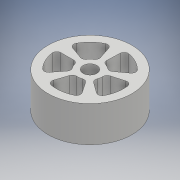
# Autodesk Inventor part: Rueda_Rin
Saved by Autodesk Inventor 2017 (Build 210142000, 142)
## iProperties
Created: 2016-07-28
Part Number: Rueda_Rin
Material: Generic
Document SubType Name: Modeling
Designer: ANDRES
Density: 1 g/cm^3
Appearance: Default
Author: ANDRES
## iProperties of the stored document Rueda_Rin_3DPrint.ipt
Created: 2016-09-14
Part Number: Rueda_Rin_3DPrint
Material: Generic
Document SubType Name: Modeling
Designer: ANDRES
Density: 1 g/cm^3
Appearance: Default
Author: ANDRES
Autodesk Inventor part; units mm, degrees
ref_plane "YZ Plane" through (0, 0, 0) normal (1, 0, 0) x (0, 1, 0)
ref_plane "XZ Plane" through (0, 0, 0) normal (0, 1, 0) x (-1, 0, 0)
ref_plane "XY Plane" through (0, 0, 0) normal (0, 0, 1) x (1, 0, 0)
sketch "Sketch4" plane through (0, 0, 0) normal (0, 0, 1) x (1, 0, 0)
  circle A0 centre (0, 0) radius 10
  arc A1 (-0.309, 0.9511) -> (-0.6428, 0.766) centre (0, 0) ccw
  line L0 (0, 0) -> (-0.309, 0.9511) construction
  line L1 (0, 0) -> (-0.9397, 0.342) construction
  arc A2 (0.5592, 0.829) -> (-0.309, 0.9511) centre (0, 0) ccw
  line L2 (-6.5104, 2.3696) -> (-2.8191, 1.0261)
  line L3 (-2.1409, 6.5891) -> (-0.9271, 2.8532)
  line L4 (-2.8191, 1.0261) -> (-6.5104, 2.3696)
  line L5 (-0.9271, 2.8532) -> (-2.1409, 6.5891)
  line L6 (-3, 0) -> (-6.9282, 0)
  arc A3 (-0.9397, 0.342) -> (-1, 0) centre (0, 0) ccw
  arc A4 (-0.309, 0.9511) -> (-0.9397, 0.342) centre (0, 0) ccw
  arc A5 (0.0349, 0.9994) -> (-0.309, 0.9511) centre (0, 0) ccw
  line L7 (0, 0) -> (0.0349, 0.9994) construction
  line L8 (0, 0) -> (-0.309, 0.9511) construction
  arc A6 (0.809, 0.5878) -> (0.0349, 0.9994) centre (0, 0) ccw
  line L9 (0, 0) -> (0.809, 0.5878) construction
  line L10 (0, 0) -> (0.0349, 0.9994) construction
  arc A7 (0.9613, 0.2756) -> (0.809, 0.5878) centre (0, 0) ccw
  line L11 (0, 0) -> (0.9613, 0.2756) construction
  line L12 (0, 0) -> (0.809, 0.5878) construction
  arc A8 (0.809, -0.5878) -> (0.9613, 0.2756) centre (0, 0) ccw
  line L13 (0, 0) -> (0.809, -0.5878) construction
  line L14 (0, 0) -> (0.9613, 0.2756) construction
  arc A9 (0.5592, -0.829) -> (0.809, -0.5878) centre (0, 0) ccw
  line L15 (0, 0) -> (0.5592, -0.829) construction
  line L16 (0, 0) -> (0.809, -0.5878) construction
  arc A10 (-0.309, -0.9511) -> (0.5592, -0.829) centre (0, 0) ccw
  line L17 (0, 0) -> (-0.309, -0.9511) construction
  line L18 (0, 0) -> (0.5592, -0.829) construction
  arc A11 (-0.6157, -0.788) -> (-0.309, -0.9511) centre (0, 0) ccw
  line L19 (0, 0) -> (-0.6157, -0.788) construction
  line L20 (0, 0) -> (-0.309, -0.9511) construction
  arc A12 (-1, 0) -> (-0.6157, -0.788) centre (0, 0) ccw
  line L21 (0.1047, 2.9982) -> (0.2418, 6.924) construction
  line L22 (-1.847, -2.364) -> (-4.2654, -5.4595) construction
  line L23 (-1.847, -2.364) -> (-4.2654, -5.4595)
  line L24 (-0.9271, -2.8532) -> (-2.1409, -6.5891)
  line L25 (1.6776, -2.4871) -> (3.8742, -5.7437)
  line L26 (2.4271, -1.7634) -> (5.605, -4.0723)
  line L27 (2.8838, 0.8269) -> (6.6598, 1.9097)
  line L28 (2.4271, 1.7634) -> (5.605, 4.0723)
  line L29 (0.1047, 2.9982) -> (0.2418, 6.924)
  arc A13 (-1.8794, 0.684) -> (-2, 0) centre (0, 0) ccw
  line L30 (0, 0) -> (0.809, 0.5878) construction
  line L31 (2.4271, 1.7634) -> (5.605, 4.0723) construction
  line L32 (0, 0) -> (-0.309, 0.9511) construction
  line L33 (-0.9271, 2.8532) -> (-2.3011, 7.0821) construction
  line L34 (0, 0) -> (0.0349, 0.9994) construction
  line L35 (0.1047, 2.9982) -> (0.2418, 6.924) construction
  line L36 (0, 0) -> (-0.309, 0.9511) construction
  line L37 (-0.9271, 2.8532) -> (-2.3011, 7.0821) construction
  line L38 (-1.6276, 0.5924) -> (-1.8794, 0.684) construction
  line L39 (-2.8191, 1.0261) -> (-6.9975, 2.5469) construction
  line L40 (0, 0) -> (-0.309, -0.9511) construction
  line L41 (-0.9271, -2.8532) -> (-2.1409, -6.5891) construction
  line L42 (0, 0) -> (0.5592, -0.829) construction
  line L43 (1.6776, -2.4871) -> (3.8742, -5.7437) construction
  line L44 (0, 0) -> (0.809, -0.5878) construction
  line L45 (2.4271, -1.7634) -> (6.0244, -4.377) construction
  line L46 (0, 0) -> (0.9613, 0.2756) construction
  line L47 (2.8838, 0.8269) -> (6.6598, 1.9097) construction
  line L48 (0, 0) -> (-0.309, -0.9511) construction
  line L49 (-0.9271, -2.8532) -> (-2.3011, -7.0821) construction
  line L50 (0, 0) -> (0.5592, -0.829) construction
  line L51 (1.5816, -2.3449) -> (3.8742, -5.7437) construction
  line L52 (0, 0) -> (0.9613, 0.2756) construction
  line L53 (2.8838, 0.8269) -> (7.1581, 2.0526) construction
  arc A14 (-1.3599, -7.8836) -> (3.4802, -7.2034) centre (0, 0) ccw
  arc A15 (-7.9179, -1.1429) -> (-5.7754, -5.5358) centre (0, 0) ccw
  arc A16 (-3.5337, 7.1773) -> (-7.0496, 3.782) centre (0, 0) ccw
  arc A17 (5.734, 5.5786) -> (1.4185, 7.8732) centre (0, 0) ccw
  arc A18 (7.0775, -3.7295) -> (7.9262, 1.0839) centre (0, 0) ccw
  arc A19 (5.605, -4.0723) -> (7.0775, -3.7295) centre (6.1928, -3.2633) ccw
  arc A20 (7.9262, 1.0839) -> (6.6598, 1.9097) centre (6.9355, 0.9484) ccw
  arc A21 (5.605, 4.0723) -> (5.734, 5.5786) centre (5.0172, 4.8813) ccw
  arc A22 (1.4185, 7.8732) -> (0.2418, 6.924) centre (1.2412, 6.8891) ccw
  arc A23 (-2.1409, 6.5891) -> (-3.5337, 7.1773) centre (-3.092, 6.2801) ccw
  arc A24 (-7.0496, 3.782) -> (-6.5104, 2.3696) centre (-6.1684, 3.3093) ccw
  arc A25 (-6.9282, 0) -> (-7.9179, -1.1429) centre (-6.9282, -1) ccw
  arc A26 (-5.7754, -5.5358) -> (-4.2654, -5.4595) centre (-5.0534, -4.8438) ccw
  arc A27 (-2.1409, -6.5891) -> (-1.3599, -7.8836) centre (-1.1899, -6.8981) ccw
  arc A28 (3.4802, -7.2034) -> (3.8742, -5.7437) centre (3.0452, -6.3029) ccw
  circle A29 centre (0, 0) radius 3
  line L54 (0, 0) -> (-0.309, 0.9511) construction
  line L55 (-0.9271, 2.8532) -> (-2.1409, 6.5891) construction
  line L56 (0, 0) -> (0.809, 0.5878) construction
  line L57 (2.4271, 1.7634) -> (5.605, 4.0723) construction
  line L58 (-0.809, 0.5878) -> (0.809, -0.5878) construction
  line L59 (2.4271, -1.7634) -> (5.605, -4.0723) construction
  point P0 (-4.5846, -5.868)
  point P1 (-1.7414, -2.2288)
  dimension "d123" = 6
  dimension "d33" = 20
  dimension "d42" = 52
  dimension "d50" = 20
  dimension "d51" = 52
  dimension "d52" = 20
  dimension "d53" = 52
  dimension "d54" = 20
  dimension "d55" = 52
  dimension "d56" = 20
  dimension "d65" = 2
  dimension "d77" = 8
  dimension "d78" = 1
  constraints: 90 end point, 41 point on circle, 21 centre point, 21 tangent, 17 point on line, 9 equal radius, 2 collinear, 1 coincident, 1 horizontal, 75 other
  measures "d33" diameter of A0
  measures "d42" angle of L0 L1
  measures "d50" angle of L7 L8
  measures "d51" angle of L9 L10
  measures "d52" angle of L11 L12
  measures "d53" angle of L13 L14
  measures "d54" angle of L15 L16
  measures "d55" angle of L17 L18
  measures "d56" angle of L19 L20
  measures "d65" radius of A13
  measures "d77" radius of A14
  measures "d78" radius of A19
extrude "Extrusion9" add sketch "Sketch4" along normal blind 8.5 contours A0 | A29
sketch "Engranaje41" plane through (0, 0, 0) normal (0, 0, -1) x (-1, 0, 0)
  circle A0 centre (0, 0) radius 1
  arc A1 (1.256, 9.9788) -> (1.0973, 10.6734) centre (-2.5912, 9.4651) ccw
  arc A2 (1.0973, 10.6734) -> (0.854, 10.6956) centre (0, 0) ccw
  arc A3 (0.854, 10.6956) -> (0.5721, 10.0412) centre (4.2626, 8.8392) ccw
  arc A4 (0.5721, 10.0412) -> (0.3434, 10.0517) centre (0, 0) ccw
  arc A5 (0.3434, 10.0517) -> (0.1221, 10.729) centre (-3.4411, 9.1902) ccw
  arc A6 (0.1221, 10.729) -> (-0.1221, 10.729) centre (0, 0) ccw
  arc A7 (-0.1221, 10.729) -> (-0.3434, 10.0517) centre (3.4411, 9.1902) ccw
  arc A8 (-0.3434, 10.0517) -> (-0.5721, 10.0412) centre (0, 0) ccw
  arc A9 (-0.5721, 10.0412) -> (-0.854, 10.6956) centre (-4.2626, 8.8392) ccw
  arc A10 (-0.854, 10.6956) -> (-1.0973, 10.6734) centre (0, 0) ccw
  arc A11 (-1.0973, 10.6734) -> (-1.256, 9.9788) centre (2.5912, 9.4651) ccw
  arc A12 (-1.256, 9.9788) -> (-1.4828, 9.9476) centre (0, 0) ccw
  arc A13 (-1.4828, 9.9476) -> (-1.8231, 10.5737) centre (-5.0487, 8.415) ccw
  arc A14 (-1.8231, 10.5737) -> (-2.0633, 10.5294) centre (0, 0) ccw
  arc A15 (-2.0633, 10.5294) -> (-2.1582, 9.8232) centre (1.7197, 9.6615) ccw
  arc A16 (-2.1582, 9.8232) -> (-2.3813, 9.7716) centre (0, 0) ccw
  arc A17 (-2.3813, 9.7716) -> (-2.777, 10.3641) centre (-5.793, 7.921) ccw
  arc A18 (-2.777, 10.3641) -> (-3.0122, 10.2982) centre (0, 0) ccw
  arc A19 (-3.0122, 10.2982) -> (-3.0425, 9.5863) centre (0.834, 9.7778) ccw
  arc A20 (-3.0425, 9.5863) -> (-3.26, 9.5145) centre (0, 0) ccw
  arc A21 (-3.26, 9.5145) -> (-3.708, 10.0686) centre (-6.4893, 7.3614) ccw
  arc A22 (-3.708, 10.0686) -> (-3.9362, 9.9816) centre (0, 0) ccw
  arc A23 (-3.9362, 9.9816) -> (-3.9017, 9.2699) centre (-0.0586, 9.8132) ccw
  arc A24 (-3.9017, 9.2699) -> (-4.1117, 9.1787) centre (0, 0) ccw
  arc A25 (-4.1117, 9.1787) -> (-4.6082, 9.6897) centre (-7.1318, 6.7408) ccw
  arc A26 (-4.6082, 9.6897) -> (-4.8276, 9.5823) centre (0, 0) ccw
  arc A27 (-4.8276, 9.5823) -> (-4.7285, 8.8767) centre (-0.9507, 9.7672) ccw
  arc A28 (-4.7285, 8.8767) -> (-4.9293, 8.7667) centre (0, 0) ccw
  arc A29 (-4.9293, 8.7667) -> (-5.4703, 9.2305) centre (-7.7153, 6.0644) ccw
  arc A30 (-5.4703, 9.2305) -> (-5.679, 9.1036) centre (0, 0) ccw
  arc A31 (-5.679, 9.1036) -> (-5.5161, 8.4099) centre (-1.8349, 9.6403) ccw
  arc A32 (-5.5161, 8.4099) -> (-5.7061, 8.2822) centre (0, 0) ccw
  arc A33 (-5.7061, 8.2822) -> (-6.287, 8.6948) centre (-8.2348, 5.3376) ccw
  arc A34 (-6.287, 8.6948) -> (-6.4833, 8.5495) centre (0, 0) ccw
  arc A35 (-6.4833, 8.5495) -> (-6.258, 7.8735) centre (-2.704, 9.4335) ccw
  arc A36 (-6.258, 7.8735) -> (-6.4356, 7.729) centre (0, 0) ccw
  arc A37 (-6.4356, 7.729) -> (-7.0516, 8.0871) centre (-8.686, 4.5667) ccw
  arc A38 (-7.0516, 8.0871) -> (-7.2338, 7.9245) centre (0, 0) ccw
  arc A39 (-7.2338, 7.9245) -> (-6.948, 7.2718) centre (-3.5506, 9.1485) ccw
  arc A40 (-6.948, 7.2718) -> (-7.1117, 7.1117) centre (0, 0) ccw
  arc A41 (-7.1117, 7.1117) -> (-7.7578, 7.4124) centre (-9.0653, 3.7579) ccw
  arc A42 (-7.7578, 7.4124) -> (-7.9245, 7.2338) centre (0, 0) ccw
  arc A43 (-7.9245, 7.2338) -> (-7.5805, 6.6098) centre (-4.3678, 8.7877) ccw
  arc A44 (-7.5805, 6.6098) -> (-7.729, 6.4356) centre (0, 0) ccw
  arc A45 (-7.729, 6.4356) -> (-8.3997, 6.6762) centre (-9.3695, 2.918) ccw
  arc A46 (-8.3997, 6.6762) -> (-8.5495, 6.4833) centre (0, 0) ccw
  arc A47 (-8.5495, 6.4833) -> (-8.1501, 5.8931) centre (-5.1488, 8.3541) ccw
  arc A48 (-8.1501, 5.8931) -> (-8.2822, 5.7061) centre (0, 0) ccw
  arc A49 (-8.2822, 5.7061) -> (-8.972, 5.8847) centre (-9.596, 2.0539) ccw
  arc A50 (-8.972, 5.8847) -> (-9.1036, 5.679) centre (0, 0) ccw
  arc A51 (-9.1036, 5.679) -> (-8.6523, 5.1276) centre (-5.8872, 7.8513) ccw
  arc A52 (-8.6523, 5.1276) -> (-8.7667, 4.9293) centre (0, 0) ccw
  arc A53 (-8.7667, 4.9293) -> (-9.4699, 5.0445) centre (-9.743, 1.1728) ccw
  arc A54 (-9.4699, 5.0445) -> (-9.5823, 4.8276) centre (0, 0) ccw
  arc A55 (-9.5823, 4.8276) -> (-9.0827, 4.3195) centre (-6.5767, 7.2834) ccw
  arc A56 (-9.0827, 4.3195) -> (-9.1787, 4.1117) centre (0, 0) ccw
  arc A57 (-9.1787, 4.1117) -> (-9.8894, 4.1624) centre (-9.8093, 0.2819) ccw
  arc A58 (-9.8894, 4.1624) -> (-9.9816, 3.9362) centre (0, 0) ccw
  arc A59 (-9.9816, 3.9362) -> (-9.4379, 3.4757) centre (-7.2118, 6.6552) ccw
  arc A60 (-9.4379, 3.4757) -> (-9.5145, 3.26) centre (0, 0) ccw
  arc A61 (-9.5145, 3.26) -> (-10.2269, 3.2459) centre (-9.7943, -0.6112) ccw
  arc A62 (-10.2269, 3.2459) -> (-10.2982, 3.0122) centre (0, 0) ccw
  arc A63 (-10.2982, 3.0122) -> (-9.7148, 2.6031) centre (-7.7871, 5.9718) ccw
  arc A64 (-9.7148, 2.6031) -> (-9.7716, 2.3813) centre (0, 0) ccw
  arc A65 (-9.7716, 2.3813) -> (-10.4797, 2.3024) centre (-9.6981, -1.4994) ccw
  arc A66 (-10.4797, 2.3024) -> (-10.5294, 2.0633) centre (0, 0) ccw
  arc A67 (-10.5294, 2.0633) -> (-9.9113, 1.7089) centre (-8.2979, 5.239) ccw
  arc A68 (-9.9113, 1.7089) -> (-9.9476, 1.4828) centre (0, 0) ccw
  arc A69 (-9.9476, 1.4828) -> (-10.6457, 1.3399) centre (-9.5216, -2.375) ccw
  arc A70 (-10.6457, 1.3399) -> (-10.6734, 1.0973) centre (0, 0) ccw
  arc A71 (-10.6734, 1.0973) -> (-10.0256, 0.8005) centre (-8.7399, 4.4627) ccw
  arc A72 (-10.0256, 0.8005) -> (-10.0412, 0.5721) centre (0, 0) ccw
  arc A73 (-10.0412, 0.5721) -> (-10.7234, 0.3663) centre (-9.2662, -3.231) ccw
  arc A74 (-10.7234, 0.3663) -> (-10.729, 0.1221) centre (0, 0) ccw
  arc A75 (-10.729, 0.1221) -> (-10.0569, -0.1145) centre (-9.1095, 3.6494) ccw
  arc A76 (-10.0569, -0.1145) -> (-10.0517, -0.3434) centre (0, 0) ccw
  arc A77 (-10.0517, -0.3434) -> (-10.7123, -0.6103) centre (-8.934, -4.0603) ccw
  arc A78 (-10.7123, -0.6103) -> (-10.6956, -0.854) centre (0, 0) ccw
  arc A79 (-10.6956, -0.854) -> (-10.0048, -1.0285) centre (-9.4036, 2.806) ccw
  arc A80 (-10.0048, -1.0285) -> (-9.9788, -1.256) centre (0, 0) ccw
  arc A81 (-9.9788, -1.256) -> (-10.6124, -1.5819) centre (-8.5277, -4.8559) ccw
  arc A82 (-10.6124, -1.5819) -> (-10.5737, -1.8231) centre (0, 0) ccw
  arc A83 (-10.5737, -1.8231) -> (-9.8698, -1.934) centre (-9.6198, 1.9392) ccw
  arc A84 (-9.8698, -1.934) -> (-9.8232, -2.1582) centre (0, 0) ccw
  arc A85 (-9.8232, -2.1582) -> (-10.4246, -2.5404) centre (-8.0508, -5.6112) ccw
  arc A86 (-10.4246, -2.5404) -> (-10.3641, -2.777) centre (0, 0) ccw
  arc A87 (-10.3641, -2.777) -> (-9.653, -2.8235) centre (-9.7563, 1.0564) ccw
  arc A88 (-9.653, -2.8235) -> (-9.5863, -3.0425) centre (0, 0) ccw
  arc A89 (-9.5863, -3.0425) -> (-10.1504, -3.4778) centre (-7.5072, -6.3201) ccw
  arc A90 (-10.1504, -3.4778) -> (-10.0686, -3.708) centre (0, 0) ccw
  arc A91 (-10.0686, -3.708) -> (-9.3563, -3.6896) centre (-9.812, 0.1648) ccw
  arc A92 (-9.3563, -3.6896) -> (-9.2699, -3.9017) centre (0, 0) ccw
  arc A93 (-9.2699, -3.9017) -> (-9.7921, -4.3865) centre (-6.9014, -6.9766) ccw
  arc A94 (-9.7921, -4.3865) -> (-9.6897, -4.6082) centre (0, 0) ccw
  arc A95 (-9.6897, -4.6082) -> (-8.982, -4.5252) centre (-9.7863, -0.7281) ccw
  arc A96 (-8.982, -4.5252) -> (-8.8767, -4.7285) centre (0, 0) ccw
  arc A97 (-8.8767, -4.7285) -> (-9.3526, -5.2587) centre (-6.2384, -7.5752) ccw
  arc A98 (-9.3526, -5.2587) -> (-9.2305, -5.4703) centre (0, 0) ccw
  arc A99 (-9.2305, -5.4703) -> (-8.5333, -5.3232) centre (-9.6795, -1.615) ccw
  arc A100 (-8.5333, -5.3232) -> (-8.4099, -5.5161) centre (0, 0) ccw
  arc A101 (-8.4099, -5.5161) -> (-8.8357, -6.0874) centre (-5.5237, -8.1111) ccw
  arc A102 (-8.8357, -6.0874) -> (-8.6948, -6.287) centre (0, 0) ccw
  arc A103 (-8.6948, -6.287) -> (-8.0139, -6.0771) centre (-9.4926, -2.4885) ccw
  arc A104 (-8.0139, -6.0771) -> (-7.8735, -6.258) centre (0, 0) ccw
  arc A105 (-7.8735, -6.258) -> (-8.2455, -6.8657) centre (-4.7632, -8.5798) ccw
  arc A106 (-8.2455, -6.8657) -> (-8.0871, -7.0516) centre (0, 0) ccw
  arc A107 (-8.0871, -7.0516) -> (-7.4281, -6.7807) centre (-9.227, -3.3414) ccw
  arc A108 (-7.4281, -6.7807) -> (-7.2718, -6.948) centre (0, 0) ccw
  arc A109 (-7.2718, -6.948) -> (-7.587, -7.587) centre (-3.9633, -8.9774) ccw
  arc A110 (-7.587, -7.587) -> (-7.4124, -7.7578) centre (0, 0) ccw
  arc A111 (-7.4124, -7.7578) -> (-6.7807, -7.4281) centre (-8.8849, -4.1666) ccw
  arc A112 (-6.7807, -7.4281) -> (-6.6098, -7.5805) centre (0, 0) ccw
  arc A113 (-6.6098, -7.5805) -> (-6.8657, -8.2455) centre (-3.1305, -9.3006) ccw
  arc A114 (-6.8657, -8.2455) -> (-6.6762, -8.3997) centre (0, 0) ccw
  arc A115 (-6.6762, -8.3997) -> (-6.0771, -8.0139) centre (-8.4692, -4.9573) ccw
  arc A116 (-6.0771, -8.0139) -> (-5.8931, -8.1501) centre (0, 0) ccw
  arc A117 (-5.8931, -8.1501) -> (-6.0874, -8.8357) centre (-2.2718, -9.5468) ccw
  arc A118 (-6.0874, -8.8357) -> (-5.8847, -8.972) centre (0, 0) ccw
  arc A119 (-5.8847, -8.972) -> (-5.3232, -8.5333) centre (-7.9833, -5.7069) ccw
  arc A120 (-5.3232, -8.5333) -> (-5.1276, -8.6523) centre (0, 0) ccw
  arc A121 (-5.1276, -8.6523) -> (-5.2587, -9.3526) centre (-1.3942, -9.7138) ccw
  arc A122 (-5.2587, -9.3526) -> (-5.0445, -9.4699) centre (0, 0) ccw
  arc A123 (-5.0445, -9.4699) -> (-4.5252, -8.982) centre (-7.4313, -6.4092) ccw
  arc A124 (-4.5252, -8.982) -> (-4.3195, -9.0827) centre (0, 0) ccw
  arc A125 (-4.3195, -9.0827) -> (-4.3865, -9.7921) centre (-0.5051, -9.8003) ccw
  arc A126 (-4.3865, -9.7921) -> (-4.1624, -9.8894) centre (0, 0) ccw
  arc A127 (-4.1624, -9.8894) -> (-3.6896, -9.3563) centre (-6.8177, -7.0584) ccw
  arc A128 (-3.6896, -9.3563) -> (-3.4757, -9.4379) centre (0, 0) ccw
  arc A129 (-3.4757, -9.4379) -> (-3.4778, -10.1504) centre (0.3881, -9.8057) ccw
  arc A130 (-3.4778, -10.1504) -> (-3.2459, -10.2269) centre (0, 0) ccw
  arc A131 (-3.2459, -10.2269) -> (-2.8235, -9.653) centre (-6.1475, -7.6492) ccw
  arc A132 (-2.8235, -9.653) -> (-2.6031, -9.7148) centre (0, 0) ccw
  arc A133 (-2.6031, -9.7148) -> (-2.5404, -10.4246) centre (1.2782, -9.7298) ccw
  arc A134 (-2.5404, -10.4246) -> (-2.3024, -10.4797) centre (0, 0) ccw
  arc A135 (-2.3024, -10.4797) -> (-1.934, -9.8698) centre (-5.4265, -8.1765) ccw
  arc A136 (-1.934, -9.8698) -> (-1.7089, -9.9113) centre (0, 0) ccw
  arc A137 (-1.7089, -9.9113) -> (-1.5819, -10.6124) centre (2.1577, -9.5732) ccw
  arc A138 (-1.5819, -10.6124) -> (-1.3399, -10.6457) centre (0, 0) ccw
  arc A139 (-1.3399, -10.6457) -> (-1.0285, -10.0048) centre (-4.6605, -8.6361) ccw
  arc A140 (-1.0285, -10.0048) -> (-0.8005, -10.0256) centre (0, 0) ccw
  arc A141 (-0.8005, -10.0256) -> (-0.6103, -10.7123) centre (3.0193, -9.3373) ccw
  arc A142 (-0.6103, -10.7123) -> (-0.3663, -10.7234) centre (0, 0) ccw
  arc A143 (-0.3663, -10.7234) -> (-0.1145, -10.0569) centre (-3.8559, -9.0241) ccw
  arc A144 (-0.1145, -10.0569) -> (0.1145, -10.0569) centre (0, 0) ccw
  arc A145 (0.1145, -10.0569) -> (0.3663, -10.7234) centre (3.8559, -9.0241) ccw
  arc A146 (0.3663, -10.7234) -> (0.6103, -10.7123) centre (0, 0) ccw
  arc A147 (0.6103, -10.7123) -> (0.8005, -10.0256) centre (-3.0193, -9.3373) ccw
  arc A148 (0.8005, -10.0256) -> (1.0285, -10.0048) centre (0, 0) ccw
  arc A149 (1.0285, -10.0048) -> (1.3399, -10.6457) centre (4.6605, -8.6361) ccw
  arc A150 (1.3399, -10.6457) -> (1.5819, -10.6124) centre (0, 0) ccw
  arc A151 (1.5819, -10.6124) -> (1.7089, -9.9113) centre (-2.1577, -9.5732) ccw
  arc A152 (1.7089, -9.9113) -> (1.934, -9.8698) centre (0, 0) ccw
  arc A153 (1.934, -9.8698) -> (2.3024, -10.4797) centre (5.4265, -8.1765) ccw
  arc A154 (2.3024, -10.4797) -> (2.5404, -10.4246) centre (0, 0) ccw
  arc A155 (2.5404, -10.4246) -> (2.6031, -9.7148) centre (-1.2782, -9.7298) ccw
  arc A156 (2.6031, -9.7148) -> (2.8235, -9.653) centre (0, 0) ccw
  arc A157 (2.8235, -9.653) -> (3.2459, -10.2269) centre (6.1475, -7.6492) ccw
  arc A158 (3.2459, -10.2269) -> (3.4778, -10.1504) centre (0, 0) ccw
  arc A159 (3.4778, -10.1504) -> (3.4757, -9.4379) centre (-0.3881, -9.8057) ccw
  arc A160 (3.4757, -9.4379) -> (3.6896, -9.3563) centre (0, 0) ccw
  arc A161 (3.6896, -9.3563) -> (4.1624, -9.8894) centre (6.8177, -7.0584) ccw
  arc A162 (4.1624, -9.8894) -> (4.3865, -9.7921) centre (0, 0) ccw
  arc A163 (4.3865, -9.7921) -> (4.3195, -9.0827) centre (0.5051, -9.8003) ccw
  arc A164 (4.3195, -9.0827) -> (4.5252, -8.982) centre (0, 0) ccw
  arc A165 (4.5252, -8.982) -> (5.0445, -9.4699) centre (7.4313, -6.4092) ccw
  arc A166 (5.0445, -9.4699) -> (5.2587, -9.3526) centre (0, 0) ccw
  arc A167 (5.2587, -9.3526) -> (5.1276, -8.6523) centre (1.3942, -9.7138) ccw
  arc A168 (5.1276, -8.6523) -> (5.3232, -8.5333) centre (0, 0) ccw
  arc A169 (5.3232, -8.5333) -> (5.8847, -8.972) centre (7.9833, -5.7069) ccw
  arc A170 (5.8847, -8.972) -> (6.0874, -8.8357) centre (0, 0) ccw
  arc A171 (6.0874, -8.8357) -> (5.8931, -8.1501) centre (2.2718, -9.5468) ccw
  arc A172 (5.8931, -8.1501) -> (6.0771, -8.0139) centre (0, 0) ccw
  arc A173 (6.0771, -8.0139) -> (6.6762, -8.3997) centre (8.4692, -4.9573) ccw
  arc A174 (6.6762, -8.3997) -> (6.8657, -8.2455) centre (0, 0) ccw
  arc A175 (6.8657, -8.2455) -> (6.6098, -7.5805) centre (3.1305, -9.3006) ccw
  arc A176 (6.6098, -7.5805) -> (6.7807, -7.4281) centre (0, 0) ccw
  arc A177 (6.7807, -7.4281) -> (7.4124, -7.7578) centre (8.8849, -4.1666) ccw
  arc A178 (7.4124, -7.7578) -> (7.587, -7.587) centre (0, 0) ccw
  arc A179 (7.587, -7.587) -> (7.2718, -6.948) centre (3.9633, -8.9774) ccw
  arc A180 (7.2718, -6.948) -> (7.4281, -6.7807) centre (0, 0) ccw
  arc A181 (7.4281, -6.7807) -> (8.0871, -7.0516) centre (9.227, -3.3414) ccw
  arc A182 (8.0871, -7.0516) -> (8.2455, -6.8657) centre (0, 0) ccw
  arc A183 (8.2455, -6.8657) -> (7.8735, -6.258) centre (4.7632, -8.5798) ccw
  arc A184 (7.8735, -6.258) -> (8.0139, -6.0771) centre (0, 0) ccw
  arc A185 (8.0139, -6.0771) -> (8.6948, -6.287) centre (9.4926, -2.4885) ccw
  arc A186 (8.6948, -6.287) -> (8.8357, -6.0874) centre (0, 0) ccw
  arc A187 (8.8357, -6.0874) -> (8.4099, -5.5161) centre (5.5237, -8.1111) ccw
  arc A188 (8.4099, -5.5161) -> (8.5333, -5.3232) centre (0, 0) ccw
  arc A189 (8.5333, -5.3232) -> (9.2305, -5.4703) centre (9.6795, -1.615) ccw
  arc A190 (9.2305, -5.4703) -> (9.3526, -5.2587) centre (0, 0) ccw
  arc A191 (9.3526, -5.2587) -> (8.8767, -4.7285) centre (6.2384, -7.5752) ccw
  arc A192 (8.8767, -4.7285) -> (8.982, -4.5252) centre (0, 0) ccw
  arc A193 (8.982, -4.5252) -> (9.6897, -4.6082) centre (9.7863, -0.7281) ccw
  arc A194 (9.6897, -4.6082) -> (9.7921, -4.3865) centre (0, 0) ccw
  arc A195 (9.7921, -4.3865) -> (9.2699, -3.9017) centre (6.9014, -6.9766) ccw
  arc A196 (9.2699, -3.9017) -> (9.3563, -3.6896) centre (0, 0) ccw
  arc A197 (9.3563, -3.6896) -> (10.0686, -3.708) centre (9.812, 0.1648) ccw
  arc A198 (10.0686, -3.708) -> (10.1504, -3.4778) centre (0, 0) ccw
  arc A199 (10.1504, -3.4778) -> (9.5863, -3.0425) centre (7.5072, -6.3201) ccw
  arc A200 (9.5863, -3.0425) -> (9.653, -2.8235) centre (0, 0) ccw
  arc A201 (9.653, -2.8235) -> (10.3641, -2.777) centre (9.7563, 1.0564) ccw
  arc A202 (10.3641, -2.777) -> (10.4246, -2.5404) centre (0, 0) ccw
  arc A203 (10.4246, -2.5404) -> (9.8232, -2.1582) centre (8.0508, -5.6112) ccw
  arc A204 (9.8232, -2.1582) -> (9.8698, -1.934) centre (0, 0) ccw
  arc A205 (9.8698, -1.934) -> (10.5737, -1.8231) centre (9.6198, 1.9392) ccw
  arc A206 (10.5737, -1.8231) -> (10.6124, -1.5819) centre (0, 0) ccw
  arc A207 (10.6124, -1.5819) -> (9.9788, -1.256) centre (8.5277, -4.8559) ccw
  arc A208 (9.9788, -1.256) -> (10.0048, -1.0285) centre (0, 0) ccw
  arc A209 (10.0048, -1.0285) -> (10.6956, -0.854) centre (9.4036, 2.806) ccw
  arc A210 (10.6956, -0.854) -> (10.7123, -0.6103) centre (0, 0) ccw
  arc A211 (10.7123, -0.6103) -> (10.0517, -0.3434) centre (8.934, -4.0603) ccw
  arc A212 (10.0517, -0.3434) -> (10.0569, -0.1145) centre (0, 0) ccw
  arc A213 (10.0569, -0.1145) -> (10.729, 0.1221) centre (9.1095, 3.6494) ccw
  arc A214 (10.729, 0.1221) -> (10.7234, 0.3663) centre (0, 0) ccw
  arc A215 (10.7234, 0.3663) -> (10.0412, 0.5721) centre (9.2662, -3.231) ccw
  arc A216 (10.0412, 0.5721) -> (10.0256, 0.8005) centre (0, 0) ccw
  arc A217 (10.0256, 0.8005) -> (10.6734, 1.0973) centre (8.7399, 4.4627) ccw
  arc A218 (10.6734, 1.0973) -> (10.6457, 1.3399) centre (0, 0) ccw
  arc A219 (10.6457, 1.3399) -> (9.9476, 1.4828) centre (9.5216, -2.375) ccw
  arc A220 (9.9476, 1.4828) -> (9.9113, 1.7089) centre (0, 0) ccw
  arc A221 (9.9113, 1.7089) -> (10.5294, 2.0633) centre (8.2979, 5.239) ccw
  arc A222 (10.5294, 2.0633) -> (10.4797, 2.3024) centre (0, 0) ccw
  arc A223 (10.4797, 2.3024) -> (9.7716, 2.3813) centre (9.6981, -1.4994) ccw
  arc A224 (9.7716, 2.3813) -> (9.7148, 2.6031) centre (0, 0) ccw
  arc A225 (9.7148, 2.6031) -> (10.2982, 3.0122) centre (7.7871, 5.9718) ccw
  arc A226 (10.2982, 3.0122) -> (10.2269, 3.2459) centre (0, 0) ccw
  arc A227 (10.2269, 3.2459) -> (9.5145, 3.26) centre (9.7943, -0.6112) ccw
  arc A228 (9.5145, 3.26) -> (9.4379, 3.4757) centre (0, 0) ccw
  arc A229 (9.4379, 3.4757) -> (9.9816, 3.9362) centre (7.2118, 6.6552) ccw
  arc A230 (9.9816, 3.9362) -> (9.8894, 4.1624) centre (0, 0) ccw
  arc A231 (9.8894, 4.1624) -> (9.1787, 4.1117) centre (9.8093, 0.2819) ccw
  arc A232 (9.1787, 4.1117) -> (9.0827, 4.3195) centre (0, 0) ccw
  arc A233 (9.0827, 4.3195) -> (9.5823, 4.8276) centre (6.5767, 7.2834) ccw
  arc A234 (9.5823, 4.8276) -> (9.4699, 5.0445) centre (0, 0) ccw
  arc A235 (9.4699, 5.0445) -> (8.7667, 4.9293) centre (9.743, 1.1728) ccw
  arc A236 (8.7667, 4.9293) -> (8.6523, 5.1276) centre (0, 0) ccw
  arc A237 (8.6523, 5.1276) -> (9.1036, 5.679) centre (5.8872, 7.8513) ccw
  arc A238 (9.1036, 5.679) -> (8.972, 5.8847) centre (0, 0) ccw
  arc A239 (8.972, 5.8847) -> (8.2822, 5.7061) centre (9.596, 2.0539) ccw
  arc A240 (8.2822, 5.7061) -> (8.1501, 5.8931) centre (0, 0) ccw
  arc A241 (8.1501, 5.8931) -> (8.5495, 6.4833) centre (5.1488, 8.3541) ccw
  arc A242 (8.5495, 6.4833) -> (8.3997, 6.6762) centre (0, 0) ccw
  arc A243 (8.3997, 6.6762) -> (7.729, 6.4356) centre (9.3695, 2.918) ccw
  arc A244 (7.729, 6.4356) -> (7.5805, 6.6098) centre (0, 0) ccw
  arc A245 (7.5805, 6.6098) -> (7.9245, 7.2338) centre (4.3678, 8.7877) ccw
  arc A246 (7.9245, 7.2338) -> (7.7578, 7.4124) centre (0, 0) ccw
  arc A247 (7.7578, 7.4124) -> (7.1117, 7.1117) centre (9.0653, 3.7579) ccw
  arc A248 (7.1117, 7.1117) -> (6.948, 7.2718) centre (0, 0) ccw
  arc A249 (6.948, 7.2718) -> (7.2338, 7.9245) centre (3.5506, 9.1485) ccw
  arc A250 (7.2338, 7.9245) -> (7.0516, 8.0871) centre (0, 0) ccw
  arc A251 (7.0516, 8.0871) -> (6.4356, 7.729) centre (8.686, 4.5667) ccw
  arc A252 (6.4356, 7.729) -> (6.258, 7.8735) centre (0, 0) ccw
  arc A253 (6.258, 7.8735) -> (6.4833, 8.5495) centre (2.704, 9.4335) ccw
  arc A254 (6.4833, 8.5495) -> (6.287, 8.6948) centre (0, 0) ccw
  arc A255 (6.287, 8.6948) -> (5.7061, 8.2822) centre (8.2348, 5.3376) ccw
  arc A256 (5.7061, 8.2822) -> (5.5161, 8.4099) centre (0, 0) ccw
  arc A257 (5.5161, 8.4099) -> (5.679, 9.1036) centre (1.8349, 9.6403) ccw
  arc A258 (5.679, 9.1036) -> (5.4703, 9.2305) centre (0, 0) ccw
  arc A259 (5.4703, 9.2305) -> (4.9293, 8.7667) centre (7.7153, 6.0644) ccw
  arc A260 (4.9293, 8.7667) -> (4.7285, 8.8767) centre (0, 0) ccw
  arc A261 (4.7285, 8.8767) -> (4.8276, 9.5823) centre (0.9507, 9.7672) ccw
  arc A262 (4.8276, 9.5823) -> (4.6082, 9.6897) centre (0, 0) ccw
  arc A263 (4.6082, 9.6897) -> (4.1117, 9.1787) centre (7.1318, 6.7408) ccw
  arc A264 (4.1117, 9.1787) -> (3.9017, 9.2699) centre (0, 0) ccw
  arc A265 (3.9017, 9.2699) -> (3.9362, 9.9816) centre (0.0586, 9.8132) ccw
  arc A266 (3.9362, 9.9816) -> (3.708, 10.0686) centre (0, 0) ccw
  arc A267 (3.708, 10.0686) -> (3.26, 9.5145) centre (6.4893, 7.3614) ccw
  arc A268 (3.26, 9.5145) -> (3.0425, 9.5863) centre (0, 0) ccw
  arc A269 (3.0425, 9.5863) -> (3.0122, 10.2982) centre (-0.834, 9.7778) ccw
  arc A270 (3.0122, 10.2982) -> (2.777, 10.3641) centre (0, 0) ccw
  arc A271 (2.777, 10.3641) -> (2.3813, 9.7716) centre (5.793, 7.921) ccw
  arc A272 (2.3813, 9.7716) -> (2.1582, 9.8232) centre (0, 0) ccw
  arc A273 (2.1582, 9.8232) -> (2.0633, 10.5294) centre (-1.7197, 9.6615) ccw
  arc A274 (2.0633, 10.5294) -> (1.8231, 10.5737) centre (0, 0) ccw
  arc A275 (1.8231, 10.5737) -> (1.4828, 9.9476) centre (5.0487, 8.415) ccw
  arc A276 (1.4828, 9.9476) -> (1.256, 9.9788) centre (0, 0) ccw
  constraints: 552 point on circle, 277 centre point
sketch "Sketch13" plane through (0, 0, 8.5) normal (0, 0, 1) x (1, 0, 0)
  line L0 (-2.8191, 1.0261) -> (-6.5104, 2.3696) projected
  arc A0 (-7.0496, 3.782) -> (-6.5104, 2.3696) centre (-6.1684, 3.3093) ccw projected
  arc A1 (-3.5337, 7.1773) -> (-7.0496, 3.782) centre (0, 0) ccw projected
  arc A2 (-2.1409, 6.5891) -> (-3.5337, 7.1773) centre (-3.092, 6.2801) ccw projected
  line L1 (-2.1409, 6.5891) -> (-0.9271, 2.8532) projected
  arc A3 (3.4802, -7.2034) -> (3.8742, -5.7437) centre (3.0452, -6.3029) ccw projected
  arc A4 (-1.3599, -7.8836) -> (3.4802, -7.2034) centre (0, 0) ccw projected
  arc A5 (-2.1409, -6.5891) -> (-1.3599, -7.8836) centre (-1.1899, -6.8981) ccw projected
  line L2 (-2.1409, -6.5891) -> (-0.9271, -2.8532) projected
  line L3 (1.6776, -2.4871) -> (3.8742, -5.7437) projected
  line L4 (-1.847, -2.364) -> (-4.2654, -5.4595) projected
  arc A6 (-5.7754, -5.5358) -> (-4.2654, -5.4595) centre (-5.0534, -4.8438) ccw projected
  arc A7 (-7.9179, -1.1429) -> (-5.7754, -5.5358) centre (0, 0) ccw projected
  arc A8 (-6.9282, 0) -> (-7.9179, -1.1429) centre (-6.9282, -1) ccw projected
  line L5 (-6.9282, 0) -> (-3, 0) projected
  line L6 (0.1047, 2.9982) -> (0.2418, 6.924) projected
  arc A9 (1.4185, 7.8732) -> (0.2418, 6.924) centre (1.2412, 6.8891) ccw projected
  arc A10 (5.734, 5.5786) -> (1.4185, 7.8732) centre (0, 0) ccw projected
  arc A11 (5.605, 4.0723) -> (5.734, 5.5786) centre (5.0172, 4.8813) ccw projected
  line L7 (5.605, 4.0723) -> (2.4271, 1.7634) projected
  line L8 (2.8838, 0.8269) -> (6.6598, 1.9097) projected
  arc A12 (7.9262, 1.0839) -> (6.6598, 1.9097) centre (6.9355, 0.9484) ccw projected
  arc A13 (7.0775, -3.7295) -> (7.9262, 1.0839) centre (0, 0) ccw projected
  arc A14 (5.605, -4.0723) -> (7.0775, -3.7295) centre (6.1928, -3.2633) ccw projected
  line L9 (5.605, -4.0723) -> (2.4271, -1.7634) projected
  circle A15 centre (0, 0) radius 1 projected
  circle A16 centre (0, 0) radius 10 projected
  arc A17 (-0.9271, 2.8532) -> (-2.8191, 1.0261) centre (0, 0) ccw projected
  arc A18 (-0.9271, -2.8532) -> (1.6776, -2.4871) centre (0, 0) ccw projected
  arc A19 (-3, 0) -> (-1.847, -2.364) centre (0, 0) ccw projected
  arc A20 (2.4271, 1.7634) -> (0.1047, 2.9982) centre (0, 0) ccw projected
  arc A21 (2.4271, -1.7634) -> (2.8838, 0.8269) centre (0, 0) ccw projected
sketch "Sketch14" plane through (0, 0, 8.5) normal (0, 0, 1) x (1, 0, 0)
  circle A0 centre (0, 0) radius 1.65
  dimension "d122" = 3.3
  constraints: 1 centre point, 1 coincident
  measures "d122" diameter of A0
fillet "Fillet12" radius 1 10 edges at (-0.9271, -2.8532, 4.25) (2.8838, 0.8269, 4.25) (2.4271, -1.7634, 4.25) (0.1047, 2.9982, 4.25) (2.4271, 1.7634, 4.25) (-0.9271, 2.8532, 4.25) (-2.8191, 1.0261, 4.25) (-3, 0, 4.25) (-1.847, -2.364, 4.25) (1.6776, -2.4871, 4.25)
extrude "Extrusion13" cut sketch "Sketch14" against normal blind 10
body "Solid2"
body "Solid3"
